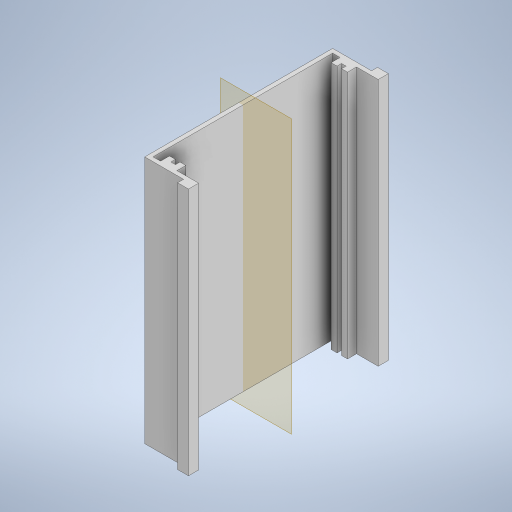
# Autodesk Inventor part: kabza başlık
Saved by Autodesk Inventor 2023 (Build 270158000, 158)
## iProperties
Created: 2023-03-22
Part Number: kabza başlık
Material: Generic
Document SubType Name: Modeling
Designer: Umut Yücesoy
Density: 1 g/cm^3
Appearance: Default
Author: Umut Yücesoy
Autodesk Inventor part; units mm, degrees
ref_plane "YZ Plane" through (0, 0, 0) normal (1, 0, 0) x (0, 1, 0)
ref_plane "XZ Plane" through (0, 0, 0) normal (0, 1, 0) x (-1, 0, 0)
sketch "Sketch1" plane through (0, 0, 0) normal (0, 1, 0) x (-1, 0, 0)
  line L0 (0, 0) -> (21.668, 0)
  line L1 (21.668, 0) -> (21.668, -61.4)
  line L2 (21.668, -61.4) -> (0, -61.4)
  line L3 (0, -61.4) -> (0, 0)
  dimension "d0" = 21.668
  dimension "d1" = 61.4
  constraints: 8 end point, 2 parallel, 1 horizontal, 1 perpendicular
  measures "d0" distance of L0.start L0.end
  measures "d1" distance of L0.end L1.end
extrude "Extrusion1" add sketch "Sketch1" along normal blind 83
sketch "Sketch2" plane through (0, 83, 0) normal (0, 1, 0) x (1, 0, 0)
  line L0 (0, 0) -> (0, 1.4)
  line L1 (0, 0) -> (0, 61.4) projected
  line L2 (0, 1.4) -> (-20.268, 1.4)
  line L3 (-21.668, 61.4) -> (-21.668, 0) projected
  line L4 (-20.268, 1.4) -> (-20.268, 61.4)
  line L5 (0, 61.4) -> (-21.668, 61.4) projected
  line L6 (-20.268, 61.4) -> (0, 61.4)
  line L7 (0, 61.4) -> (0, 1.4)
  line L8 (-21.668, 61.4) -> (0, 61.4)
  line L9 (0, 61.4) -> (0, 62.8)
  line L10 (0, 62.8) -> (-21.668, 62.8)
  line L11 (-21.668, 62.8) -> (-21.668, 61.4)
  dimension "d4" = 1.4
  dimension "d5" = 20.268
  dimension "d6" = 1.4
  constraints: 18 end point, 4 perpendicular, 3 parallel, 1 horizontal, 1 point on line
  measures "d4" distance of L0.start L0.end
  measures "d5" distance of L0.end L2.end
  measures "d6" distance of L9.end L8.end
extrude "Extrusion2" add sketch "Sketch2" against normal blind 83 contours L5 L11 L10 L9
sketch "Sketch3" plane through (0, 83, 0) normal (0, 1, 0) x (1, 0, 0)
  line L0 (0, 0) -> (0, 62.8) projected
  line L1 (0, 0) -> (0, 1.4)
  line L2 (0, 1.4) -> (-20.268, 1.4)
  line L3 (-20.268, 1.4) -> (-20.268, 61.4)
  line L4 (-21.668, 62.8) -> (-21.668, 0) projected
  line L5 (-20.268, 61.4) -> (0, 61.4)
  dimension "d9" = 1.4
  dimension "d10" = 20.268
  dimension "d11" = 60
  constraints: 8 end point, 2 perpendicular, 2 point on line, 1 parallel
  measures "d9" distance of L0.start L1.end
  measures "d10" distance of L1.end L2.end
  measures "d11" distance of L2.end L3.end
extrude "Extrusion3" cut sketch "Sketch3" against normal blind 129.5
sketch "Sketch4" plane through (0, 83, 0) normal (0, 1, 0) x (1, 0, 0)
  line L0 (0, 0) -> (0, 1.4) projected
  line L1 (0, 0) -> (0, -2)
  line L2 (0, -2) -> (-3.619, -2)
  line L3 (-20.268, 1.4) -> (0, 1.4) projected
  line L4 (-3.619, -2) -> (-3.619, 0)
  line L5 (-21.668, 0) -> (0, 0) projected
  line L6 (-3.619, 0) -> (-7.238, 0)
  line L7 (-7.238, 0) -> (-7.238, 1.4)
  line L8 (-7.238, 1.4) -> (-7.238, 4.4)
  line L9 (-7.238, 4.4) -> (-9.238, 4.4)
  line L10 (-9.238, 4.4) -> (-9.238, 2.9)
  line L11 (-9.238, 2.9) -> (-10.738, 2.9)
  line L12 (-10.738, 2.9) -> (-10.738, 4.4)
  line L13 (-10.738, 4.4) -> (-12.738, 4.4)
  line L14 (-12.738, 4.4) -> (-12.738, 1.4)
  dimension "d14" = 2
  dimension "d15" = 3.619
  dimension "d16" = 3.619
  dimension "d17" = 3
  dimension "d18" = 2
  dimension "d19" = 1.5
  dimension "d20" = 1.5
  dimension "d21" = 2
  constraints: 24 end point, 5 point on line, 4 perpendicular, 3 vertical, 1 horizontal, 3 other
  measures "d14" distance of L0.start L1.end
  measures "d15" distance of L1.end L2.end
  measures "d16" distance of L4.end L6.end
  measures "d17" distance of L7.end L8.end
  measures "d18" distance of L8.end L9.end
  measures "d19" distance of L10.end L11.end
  measures "d20" distance of L11.end L12.end
  measures "d21" distance of L12.end L13.end
extrude "Extrusion4" add sketch "Sketch4" against normal blind 83 contours L3 L14 L13 L12 L11 L10 L9 L8 | L1 L2 L4 L5
ref_plane "Work Plane1" through (0, 0, -31.4) normal (0, 0, 1) x (1, 0, 0)
mirror "Mirror1" about plane through (0, 0, -31.4) normal (0, 0, 1) of "Extrusion4"
sketch "Sketch5" plane through (-21.668, 0, 0) normal (-1, 0, 0) x (0, 0, 1)
  line L0 (-62.8, 83) -> (-62.8, 0) projected
  line L1 (0, 0) -> (-62.8, 0)
  line L2 (-62.8, 0) -> (-62.8, 83)
  line L3 (-62.8, 83) -> (0, 83)
  line L4 (0, 83) -> (0, 0)
  constraints: 8 end point, 2 parallel, 1 horizontal, 1 perpendicular
extrude "Extrusion5" cut sketch "Sketch5" against normal blind 6.454
sketch "Sketch6" plane through (-15.214, 0, 0) normal (-1, 0, 0) x (0, 0, 1)
  line L0 (2, 0) -> (0, 0) projected
  line L1 (-62.8, 83) -> (-61.4, 83) projected
  line L2 (0, 0) -> (-62.8, 0)
  line L3 (-62.8, 0) -> (-62.8, 83)
  line L4 (-62.8, 83) -> (0, 83)
  line L5 (0, 83) -> (0, 0)
  constraints: 8 end point, 2 parallel, 1 horizontal, 1 perpendicular
extrude "Extrusion6" add sketch "Sketch6" along normal blind 1.4
body "Solid1"
